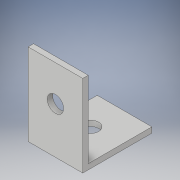
# Autodesk Inventor part: Fixador acelerometro dianteiro
Saved by Autodesk Inventor 2019 (Build 230136000, 136)
## iProperties
Created: 2021-05-27
Part Number: Fixador acelerometro dianteiro
Material: Generic
Document SubType Name: Modeling
Designer: hoope
Density: 1 g/cm^3
Appearance: Default
Author: hoope
Autodesk Inventor part; units mm, degrees
ref_plane "YZ Plane" through (0, 0, 0) normal (1, 0, 0) x (0, 1, 0)
ref_plane "XZ Plane" through (0, 0, 0) normal (0, 1, 0) x (-1, 0, 0)
ref_plane "XY Plane" through (0, 0, 0) normal (0, 0, 1) x (1, 0, 0)
sketch "Esboço1" plane through (0, 0, 0) normal (0, 0, 1) x (1, 0, 0)
  line L0 (0, 0) -> (20, 0)
  line L1 (20, 0) -> (20, 2)
  line L2 (20, 2) -> (0, 2)
  line L3 (0, 2) -> (0, 0)
  dimension "d0" = 20
  dimension "d1" = 2
  constraints: 8 end point, 2 parallel, 1 horizontal, 1 perpendicular
  measures "d0" distance of L2.end L1.end
  measures "d1" distance of L1.end L0.end
extrude "Extrusão1" add sketch "Esboço1" along normal blind 25.3
sketch "Esboço2" plane through (0, 2, 0) normal (0, 1, 0) x (1, 0, 0)
  line L0 (0, -25.3) -> (20, -25.3) projected
  line L1 (0, 0) -> (0, -25.3) projected
  line L2 (20, -25.3) -> (0, -25.3)
  line L3 (0, -25.3) -> (0, -23.3)
  line L4 (0, -23.3) -> (20, -23.3)
  line L5 (20, -23.3) -> (20, -25.3)
  dimension "d4" = 2
  constraints: 8 end point, 2 parallel, 1 horizontal, 1 perpendicular, 1 point on line
  measures "d4" distance of L2.end L3.end
extrude "Extrusão2" add sketch "Esboço2" along normal blind 28
sketch "Esboço3" plane through (0, 2, 0) normal (0, 1, 0) x (1, 0, 0)
  circle A0 centre (8.75, -11.25) radius 3
  line L0 (20, 0) -> (0, 0) projected
  line L1 (0, 0) -> (0, -23.3) projected
  dimension "d7" = 6
  dimension "d8" = 11.25
  dimension "d9" = 8.75
  constraints: 1 centre point
  measures "d7" diameter of A0
  measures "d8" distance from line of L0 A0.centre
  measures "d9" distance from line of L1 A0.centre
extrude "Extrusão3" cut sketch "Esboço3" against normal blind 28
sketch "Esboço4" plane through (20, 2, 23.3) normal (0, 0, -1) x (-1, 0, 0)
  circle A0 centre (10, 14.93) radius 3
  line L0 (20, 0) -> (20, 28) projected
  line L1 (0, 28) -> (20, 28) projected
  point P0 (20, -2)
  dimension "d12" = 6
  dimension "d13" = 10
  dimension "d14" = 13.07
  constraints: 1 centre point
  measures "d12" diameter of A0
  measures "d13" distance from line of L0 A0.centre
  measures "d14" distance from line of L1 A0.centre
extrude "Extrusão4" cut sketch "Esboço4" against normal blind 28
